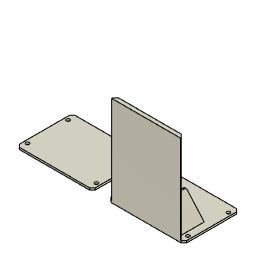
CPU Tray - Template V3 (Autodesk Fusion 360 design; units mm, degrees)
Autodesk Fusion 360 part; units mm, degrees
sketch "Sketch1" plane through (0, 0, 0) normal (0, 0, 1) x (1, 0, 0)
  circle A0 centre (-75.25, 8) radius 1.4
  circle A1 centre (-75.25, 8) radius 2.5
  line L0 (-3.75, 1) -> (-3.75, 8) construction
  line L1 (-7.5, 29) -> (0, 29) construction
  line L2 (-7.5, 0) -> (-71.5, 0)
  line L3 (-75.25, 1) -> (-71.5, 4.75)
  line L4 (-7.5, 0) -> (-7.5, 58)
  circle A2 centre (-75.25, 50) radius 2.5
  line L5 (-79, 55) -> (-79, 3)
  line L6 (-7.5, 0) -> (-3, 0)
  line L7 (-7.5, 58) -> (-3, 58)
  line L8 (-3.75, 0) -> (-3.75, 1)
  circle A3 centre (-3.75, 50) radius 1.4
  line L9 (-3, 58) -> (0, 55)
  line L10 (-76, 58) -> (-79, 55)
  line L11 (-75.25, 0) -> (-75.25, 1)
  circle A4 centre (-3.75, 8) radius 1.4
  line L12 (-7.5, 0) -> (-7.5, 58)
  line L13 (-7.5, 58) -> (-76, 58)
  circle A5 centre (-3.75, 8) radius 2.5
  line L14 (-71.5, 58) -> (-71.5, 0)
  line L15 (-3.75, 1) -> (-7.5, 4.75)
  line L16 (-76, 0) -> (-71.5, 0)
  line L17 (0, 3) -> (0, 55)
  line L18 (-76, 0) -> (-79, 3)
  line L19 (-39.5, 0) -> (-39.5, 27) construction
  circle A6 centre (-3.75, 50) radius 2.5
  circle A7 centre (-75.25, 50) radius 1.4
  line L20 (-3, 0) -> (0, 3)
  point P0 (-79, 0)
  point P1 (7.1, -7)
  point P2 (0, 58)
  dimension "d1" = 7.5
  dimension "d2" = 3
  dimension "d3" = 3
  dimension "d4" = 135
  dimension "d5" = 1
  dimension "d6" = 5
  dimension "d7" = 2.8
  dimension "d8" = 3
  dimension "d9" = 3
  dimension "d10" = 3
  dimension "d11" = 3
  dimension "d12" = 8
  dimension "d13" = 7.5
  dimension "d14" = 64
  dimension "d15" = 3.75
  dimension "d16" = 3
  dimension "d17" = 3
  constraint perpendicular L12 L13
  constraint perpendicular L2 L5
  constraint perpendicular L6 L12
  constraint perpendicular L7 L17
  constraint coincident P2 L7
  constraint coincident P2 L17
  constraint perpendicular L2 L14
  constraint coincident L14.start L13
  constraint perpendicular L6 L8
  constraint coincident L15.end L4
  constraint parallel L0 L8
  constraint coincident L0.end A4.centre
  constraint coincident L8.start L6
  constraint coincident origin L6
  constraint coincident origin L17
  constraint coincident P0 L2
  constraint coincident P0 L5
  constraint midpoint L1.start L12
  constraint perpendicular L1 L12
  constraint symmetric L1 A5 A6
  constraint symmetric L1 A3 A4
  constraint perpendicular L14 L16
  constraint midpoint L19.start L2
  constraint perpendicular L2 L19
  constraint symmetric L8.start L11.start L19
  constraint symmetric L0.start L3.start L19
  constraint symmetric L15.end L3.end L19
  constraint symmetric A1 A5 L19
  constraint symmetric A0 A4 L19
  constraint symmetric A2 L19 A6
  constraint symmetric A3 L19 A7
  constraint coincident L1.end L17
  measures "d1" distance of origin L2.start
  measures "d2" distance of P2 L7.end
  measures "d3" distance of P2 L9.end
  measures "d4" angle of L8 L15
  measures "d5" distance of L8.start L0.start
  measures "d6" diameter of A5
  measures "d7" diameter of A4
  measures "d8" distance of L6.end origin
  measures "d9" distance of L17.start origin
  measures "d10" distance of P0 L16.start
  measures "d11" distance of P0 L5.end
  measures "d12" distance of L0.end L6
  measures "d13" distance of L5 L14
  measures "d14" distance of L12 L14
  measures "d15" distance of L0 L17
  measures "d16" horizontal distance of L10.start L5.start
  measures "d17" vertical distance of L10.start L5.start
sketch "Sketch2" plane through (0, 0, 0) normal (0, 0, 1) x (1, 0, 0)
  line L0 (-7.5, 58) -> (-76, 58) construction
  line L1 (-76, 58) -> (-79, 55)
  line L2 (-79, 55) -> (-79, 3)
  line L3 (-76, 0) -> (-79, 3)
  line L4 (-76, 0) -> (-71.5, 0)
  line L5 (-7.5, 0) -> (-3, 0)
  line L6 (-3, 0) -> (0, 3)
  line L7 (-3, 58) -> (0, 55)
  line L8 (-7.5, 58) -> (-3, 58) construction
  line L9 (0, 3) -> (0, 55)
  line L10 (-7.5, 0) -> (-71.5, 0)
  line L11 (-7.5, 57.8) -> (-75.9172, 57.8)
  line L12 (-75.9172, 57.8) -> (-78.8, 54.9172)
  line L13 (-78.8, 54.9172) -> (-78.8, 3.0828)
  line L14 (-75.9172, 0.2) -> (-78.8, 3.0828)
  line L15 (-75.9172, 0.2) -> (-71.5, 0.2)
  line L16 (-7.5, 0.2) -> (-71.5, 0.2)
  line L17 (-7.5, 0.2) -> (-3.0828, 0.2)
  line L18 (-3.0828, 0.2) -> (-0.2, 3.0828)
  line L19 (-0.2, 3.0828) -> (-0.2, 54.9172)
  line L20 (-3.0828, 57.8) -> (-0.2, 54.9172)
  line L21 (-7.5, 57.8) -> (-3.0828, 57.8)
  dimension "d19" = -0.2
sketch "Sketch3" plane through (0, 0, 0) normal (0, 0, 1) x (1, 0, 0)
  line L0 (-71.5, 58) -> (-71.5, 0) construction
  line L1 (-7.5, 0) -> (-7.5, 58) construction
  line L2 (-78.8, 54.9172) -> (-78.8, 3.0828)
  line L3 (-75.9172, 0.2) -> (-78.8, 3.0828)
  line L4 (-75.9172, 0.2) -> (-71.5, 0.2)
  line L5 (-7.5, 0.2) -> (-71.5, 0.2)
  line L6 (-7.5, 0.2) -> (-3.0828, 0.2)
  line L7 (-3.0828, 0.2) -> (-0.2, 3.0828)
  line L8 (-0.2, 3.0828) -> (-0.2, 54.9172)
  line L9 (-3.0828, 57.8) -> (-0.2, 54.9172)
  line L10 (-7.5, 57.8) -> (-3.0828, 57.8)
  line L11 (-7.5, 57.8) -> (-75.9172, 57.8)
  line L12 (-75.9172, 57.8) -> (-78.8, 54.9172)
  line L13 (-71.1, 58) -> (-71.1, 0)
  line L14 (-39.5, 0.2) -> (-39.5, 13) construction
  line L15 (-7.9, 58) -> (-7.9, 0)
  circle A0 centre (-75.25, 50) radius 1.4 construction
  circle A1 centre (-75.25, 8) radius 1.4 construction
  circle A2 centre (-75.25, 50) radius 1.8
  circle A3 centre (-75.25, 8) radius 1.8
  circle A4 centre (-3.75, 8) radius 1.8
  circle A5 centre (-3.75, 50) radius 1.8
  line L16 (-69.5, 58) -> (-69.5, 0)
  line L17 (-9.5, 58) -> (-9.5, 0)
  line L18 (-9.5, 4.2) -> (-69.5, 4.2)
  line L19 (-75.25, 0) -> (-75.25, 1) construction
  line L20 (-75.25, 1) -> (-71.5, 4.75) construction
  line L21 (-75.25, 1) -> (-71.1, 5.15)
  line L22 (-75.25, 1) -> (-75.25, 0.2)
  line L23 (-3.75, 1) -> (-3.75, 0.2)
  line L24 (-3.75, 1) -> (-7.9, 5.15)
  line L25 (-69.5, 4.2) -> (-72.05, 4.2)
  line L26 (-9.5, 4.2) -> (-6.95, 4.2)
  line L27 (-7.9, 29) -> (-9.5, 29)
  line L28 (-71.1, 29) -> (-69.5, 29)
  dimension "d20" = -0.4
  dimension "d21" = 3.6
  dimension "d22" = 3.6
  dimension "d23" = -2
  dimension "d31" = 4
  constraint midpoint L5 L14.start
  constraint perpendicular L5 L14
  constraint symmetric L13.start L14 L15.start
  constraint symmetric L13.end L14 L15.end
  constraint concentric A0 A2
  constraint concentric A1 A3
  constraint symmetric L14 A2 A5
  constraint symmetric L14 A3 A4
  constraint symmetric L14 L16.start L17.start
  constraint symmetric L14 L16.end L17.end
  constraint coincident L16 L18.end
  constraint coincident L17 L18.start
  constraint coincident L19.end L20.start
  constraint coincident L13 L21.end
  constraint parallel L20 L21
  constraint coincident L19 L22.end
  constraint coincident L4 L22.end
  constraint symmetric L14 L19.end L23.start
  constraint symmetric L14 L21.end L24.end
  constraint symmetric L14 L22.end L23.end
  constraint coincident L21 L25.end
  constraint horizontal L25
  constraint symmetric L14 L18.end L18.start
  constraint symmetric L14 L25.end L26.end
  constraint midpoint L15 L27.start
  constraint midpoint L17 L27.end
  constraint perpendicular L17 L27
  constraint symmetric L14 L27.start L28.start
  constraint symmetric L14 L27.end L28.end
  measures "d21" diameter of A2
  measures "d22" diameter of A3
  measures "d31" distance of L5 L18
extrude "Extrude1" add sketch "Sketch3" against normal blind 2 makes body 1 in component "Panel Template"
extrude "Extrude1'" add sketch "Sketch3" against normal blind 2 separate body makes body 2 in component "Tray Template"
extrude "Extrude2" add sketch "Sketch3" along normal blind 91.9 contours L4 L5 L13 L21 L22 L25 | L5 L13 L16 L25 | L5 L16 L17 L18 | L5 L15 L17 L26 | L5 L6 L15 L23 L24 L26 bodies 2 in component "Tray Template"
extrude "Extrude3" add sketch "Sketch3" along normal blind 40 contours L13 L16 L25 L28 | L15 L17 L26 L27 bodies 2 in component "Tray Template"
draft "Draft1" angle 25 neutral plane through (0, 0, 0) pull (0, 0, 1) 2 faces at (-8.4333, 29, 13.3333) (-70.5667, 29, 13.3333) on bodies 2 in component "Tray Template"
fillet "Fillet1" radius 3 3 edges at (-8.7, 10.3477, 40) (-70.3, 10.3477, 40) (-70.3, 29, 0) on bodies 2 in component "Tray Template"
fillet "Fillet2" radius 0.5 2 edges at (-9.5, 4.2, 20) (-69.5, 4.2, 20) on bodies 2 in component "Tray Template"
fillet "Fillet3" radius 0.6 5 edges at (-69.5, 17.8056, 0) (-69.3536, 4.3464, 0) (-39.5, 4.2, 0) (-9.6464, 4.3464, 0) (-9.5, 16.85, 0) on bodies 2 in component "Tray Template"
component "Panel Template" placed x (1, 0, 0) y (0, 1, 0) z (0, 0, 1) at (-95, 0, 0)
component "Tray Template" placed x (1, 0, 0) y (0, 1, 0) z (0, 0, 1) at (0, 0, 0)
equation "d22 = d21"
